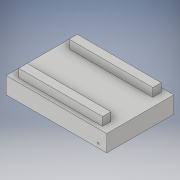
# Autodesk Inventor part: BS #3
Saved by Autodesk Inventor 2019 (Build 230136000, 136)
## iProperties
Created: 2019-02-18
Part Number: BS #3
Material: Generic
Document SubType Name: Modeling
Designer: Tesler
Density: 1 g/cm^3
Appearance: Default
Author: Tesler
Autodesk Inventor part; units mm, degrees
ref_plane "YZ Plane" through (0, 0, 0) normal (1, 0, 0) x (0, 1, 0)
ref_plane "XZ Plane" through (0, 0, 0) normal (0, 1, 0) x (-1, 0, 0)
sketch "Sketch1" plane through (0, 0, 0) normal (0, 1, 0) x (-1, 0, 0)
  line L0 (0, 0) -> (152.4, 0)
  line L1 (152.4, 0) -> (152.4, -101.6)
  line L2 (152.4, -101.6) -> (0, -101.6)
  line L3 (0, -101.6) -> (0, 0)
  dimension "d0" = 152.4
  dimension "d1" = 101.6
  constraints: 8 end point, 2 parallel, 1 horizontal, 1 perpendicular
  measures "d0" distance of L1.end L2.end
  measures "d1" distance of L0.end L1.end
extrude "Extrusion1" add sketch "Sketch1" along normal blind 38.1
ref_plane "Work Plane1" through (-152.4, 0, -50.8) normal (0, 0, 1) x (1, 0, 0)
sketch "Sketch3" plane through (0, 38.1, 0) normal (0, 1, 0) x (1, 0, 0)
  line L0 (-139.7, 95.25) -> (-12.7, 95.25)
  line L1 (-12.7, 95.25) -> (-12.7, 82.55)
  line L2 (-12.7, 82.55) -> (-139.7, 82.55)
  line L3 (-139.7, 82.55) -> (-139.7, 95.25)
  line L4 (0, 101.6) -> (-152.4, 101.6) projected
  line L5 (0, 0) -> (0, 101.6) projected
  line L6 (-152.4, 101.6) -> (-152.4, 0) projected
  line L7 (30.48, 50.8) -> (-182.88, 50.8) projected
  line L8 (-139.7, 6.35) -> (-12.7, 6.35)
  line L9 (-12.7, 6.35) -> (-12.7, 19.05)
  line L10 (-12.7, 19.05) -> (-139.7, 19.05)
  line L11 (-139.7, 19.05) -> (-139.7, 6.35)
  line L12 (0, 101.6) -> (-152.4, 101.6)
  line L13 (-152.4, 101.6) -> (-152.4, 0)
  line L14 (-152.4, 0) -> (0, 0)
  line L15 (0, 0) -> (0, 101.6)
  dimension "d12" = 6.35
  dimension "d13" = 12.7
  dimension "d14" = 12.7
  dimension "d15" = 12.7
  constraints: 24 end point, 4 parallel, 4 symmetric about line, 2 horizontal, 2 perpendicular
  measures "d12" distance between parallel lines of L0 L4
  measures "d13" distance between parallel lines of L5 L1
  measures "d14" distance between parallel lines of L6 L3
  measures "d15" distance between parallel lines of L0 L2
extrude "Extrusion3" cut sketch "Sketch3" against normal blind 12.7
sketch "Sketch4" plane through (0, 0, -101.6) normal (0, 0, -1) x (-1, 0, 0)
  line L0 (0, 0) -> (0, 25.4) projected
  line L1 (152.4, 0) -> (0, 0) projected
  point P0 (12.7, 6.35)
  dimension "d18" = 12.7
  dimension "d19" = 6.35
  measures "d18" distance from line of L0 point (12.7, 6.35)
  measures "d19" distance from line of L1 point (12.7, 6.35)
hole "Hole1" at (-12.7, 6.35, -101.6) direction (0, 0, 1) diameter 2.54 end through all
body "Solid1"
